Autodesk Fusion 360 part; units mm, degrees
(part 2 of 2)
  arc A365 (-6.1668, -296.7812) -> (-6.5328, -295.4151) centre (-7.0328, -296.2812) ccw
  arc A366 (-3.876, -300.2037) -> (-3.3, -299.7095) centre (-3.8, -299.7095) ccw
  line L347 (-6.6168, -297.5606) -> (-6.1668, -296.7812)
  arc A367 (-2.3, -290.7464) -> (-3.3, -291.7464) centre (-2.3, -291.7464) ccw
  line L348 (-3.6, -298.8464) -> (-4.55, -298.8464)
  arc A368 (-7.4653, -294.5303) -> (-7.3555, -294.9401) centre (-7.2055, -294.6803) ccw
  arc A369 (-5.55, -297.8464) -> (-4.55, -298.8464) centre (-4.55, -297.8464) ccw
  line L349 (-3.3, -291.7464) -> (-3.3, -295.7464)
  line L350 (-3.3, -299.1464) -> (-3.3, -299.7095)
  arc A370 (3.3, -291.7464) -> (2.3, -290.7464) centre (2.3, -291.7464) ccw
  line L351 (2.3, -290.7464) -> (-2.3, -290.7464)
  arc A371 (-3.6, -296.0464) -> (-3.3, -295.7464) centre (-3.6, -295.7464) ccw
  line L352 (-3.3, -299.1464) -> (-3.3, -295.7464)
  line L353 (3.3, -299.1464) -> (3.3, -299.7095)
  arc A372 (-5.5153, -291.1528) -> (-5.8814, -289.7868) centre (-6.3814, -290.6528) ccw
  arc A373 (-20.5017, -281.5828) -> (-21.8678, -281.2168) centre (-21.3678, -282.0828) ccw
  arc A374 (-23.8464, -279.55) -> (-22.8464, -280.55) centre (-22.8464, -279.55) ccw
  line L354 (-3.3, -254.3536) -> (-3.3, -258.2536)
  arc A375 (-3.3, -258.2536) -> (-2.3, -259.2536) centre (-2.3, -258.2536) ccw
  line L355 (-3.6, -251.1536) -> (-4.55, -251.1536)
  arc A376 (-23.765, -284.2451) -> (-23.0491, -284.4969) centre (-23.2991, -284.0639) ccw
  line L356 (3.3, -250.8536) -> (3.3, -250.2905)
  arc A377 (-5.8814, -260.2132) -> (-5.5153, -258.8472) centre (-6.3814, -259.3472) ccw
  line L357 (3.3, -258.2536) -> (3.3, -254.2536)
  arc A378 (-6.5828, -254.4983) -> (-6.2168, -253.1322) centre (-7.0828, -253.6322) ccw
  line L358 (-6.2168, -253.1322) -> (-6.6168, -252.4394)
  line L359 (-2.3, -259.2536) -> (2.3, -259.2536)
  arc A379 (3.3, -250.8536) -> (3.6, -251.1536) centre (3.6, -250.8536) ccw
  arc A380 (3.3, -299.7095) -> (3.876, -300.2037) centre (3.8, -299.7095) ccw
  line L360 (3.3, -250.8536) -> (3.3, -254.2536)
  line L361 (-7.4055, -254.9733) -> (-6.5828, -254.4983)
  arc A381 (-7.4055, -254.9733) -> (-7.5153, -255.3831) centre (-7.2555, -255.2331) ccw
  arc A382 (-3.6, -251.1536) -> (-3.3, -250.8536) centre (-3.6, -250.8536) ccw
  arc A383 (-4.55, -251.1536) -> (-5.55, -252.1536) centre (-4.55, -252.1536) ccw
  arc A384 (-3.3, -254.3536) -> (-3.6, -254.0536) centre (-3.6, -254.3536) ccw
  line L362 (-4.55, -254.0536) -> (-3.6, -254.0536)
  arc A385 (3.6, -253.9536) -> (3.3, -254.2536) centre (3.6, -254.2536) ccw
  line L363 (-3.3, -250.8536) -> (-3.3, -250.2905)
  line L364 (-17.0106, -291.2297) -> (-16.2312, -290.7797)
  arc A386 (-16.2297, -292.0106) -> (-15.8636, -293.3766) centre (-15.3636, -292.5106) ccw
  line L365 (-16.1528, -280.5153) -> (-19.6169, -282.5153)
  line L366 (-20.0267, -282.4055) -> (-20.5017, -281.5828)
  line L367 (-9.2153, -297.5614) -> (-9.4969, -298.0491)
  arc A387 (-19.889, -290.9586) -> (-15.9586, -294.889) centre (0, -275) ccw
  line L368 (-12.4868, -284.8651) -> (-14.7868, -280.8814)
  line L369 (-20.9464, -279.55) -> (-20.9464, -278.6)
  line L370 (-13.6409, -291.4268) -> (-14.4636, -290.9518)
  arc A388 (-22.5606, -281.6168) -> (-22.9266, -282.9828) centre (-22.0606, -282.4828) ccw
  arc A389 (-21.9464, -280.55) -> (-20.9464, -279.55) centre (-21.9464, -279.55) ccw
  line L371 (-24.1464, -278.3) -> (-20.6464, -278.3)
  arc A390 (-14.9311, -294.2614) -> (-15.0409, -293.8516) centre (-15.1909, -294.1114) ccw
  line L372 (-14.9311, -294.2614) -> (-13.2311, -291.3169)
  line L373 (-22.8464, -280.55) -> (-21.9464, -280.55)
  arc A391 (-19.7491, -290.2126) -> (-19.889, -290.9586) centre (-19.4991, -290.6457) ccw
  arc A392 (-13.6409, -291.4268) -> (-13.2311, -291.3169) centre (-13.4909, -291.1669) ccw
  arc A393 (-9.4969, -298.0491) -> (-9.2451, -298.765) centre (-9.0639, -298.2991) ccw
  arc A394 (-15.9586, -294.889) -> (-15.2126, -294.7491) centre (-15.6457, -294.4991) ccw
  line L374 (-16.2303, -288.1811) -> (-12.8528, -286.2311)
  arc A395 (-8.8055, -297.4516) -> (-9.2153, -297.5614) centre (-8.9555, -297.7114) ccw
  line L375 (-19.2614, -289.9311) -> (-19.7491, -290.2126)
  line L376 (-15.8297, -291.3178) -> (-16.2297, -292.0106)
  line L377 (-11.2311, -287.8528) -> (-13.2311, -291.3169)
  line L378 (-18.8516, -290.0409) -> (-18.3766, -290.8636)
  line L379 (-14.9311, -294.2614) -> (-15.2126, -294.7491)
  arc A396 (-18.3766, -290.8636) -> (-17.0106, -291.2297) centre (-17.5106, -290.3636) ccw
  arc A397 (-14.4636, -290.9518) -> (-15.8297, -291.3178) centre (-14.9636, -291.8178) ccw
  arc A398 (-16.2312, -290.7797) -> (-15.8651, -289.4136) centre (-16.7312, -289.9136) ccw
  arc A399 (-9.8651, -287.4868) -> (-11.2311, -287.8528) centre (-10.3651, -288.3528) ccw
  arc A400 (-16.2303, -288.1811) -> (-16.3401, -288.5909) centre (-16.0803, -288.4409) ccw
  line L380 (-15.0409, -293.8516) -> (-15.8636, -293.3766)
  line L381 (-15.8651, -289.4136) -> (-16.3401, -288.5909)
  arc A401 (-18.8516, -290.0409) -> (-19.2614, -289.9311) centre (-19.1114, -290.1909) ccw
  line L382 (-19.2614, -289.9311) -> (-16.2303, -288.1811)
  line L383 (-20.4151, -268.4672) -> (-19.9401, -267.6445)
  line L384 (-23.8464, -271.4) -> (-23.8464, -270.45)
  line L385 (-22.0464, -269.45) -> (-22.8464, -269.45)
  arc A402 (-22.9266, -267.0172) -> (-22.5606, -268.3832) centre (-22.0606, -267.5172) ccw
  arc A403 (-21.7812, -268.8332) -> (-20.4151, -268.4672) centre (-21.2812, -267.9672) ccw
  line L386 (-14.7868, -269.1186) -> (-12.4868, -265.1349)
  arc A404 (-19.5303, -267.5347) -> (-19.9401, -267.6445) centre (-19.6803, -267.7945) ccw
  arc A405 (-22.4516, -266.1945) -> (-22.5614, -265.7847) centre (-22.7114, -266.0445) ccw
  arc A406 (-12.4868, -265.1349) -> (-12.8528, -263.7689) centre (-13.3528, -264.6349) ccw
  line L387 (-19.5303, -267.5347) -> (-16.1528, -269.4847)
  arc A407 (-21.0464, -270.45) -> (-22.0464, -269.45) centre (-22.0464, -270.45) ccw
  line L388 (-24.1464, -271.7) -> (-24.7095, -271.7)
  line L389 (-22.5606, -268.3832) -> (-21.7812, -268.8332)
  line L390 (-22.4516, -266.1945) -> (-22.9266, -267.0172)
  line L391 (-24.1464, -271.7) -> (-20.7464, -271.7)
  arc A408 (-23.765, -265.7549) -> (-25.2037, -271.124) centre (0, -275) ccw
  arc A409 (-16.1528, -269.4847) -> (-14.7868, -269.1186) centre (-15.6528, -268.6186) ccw
  line L392 (-16.7464, -271.7) -> (-20.7464, -271.7)
  arc A410 (-22.8464, -269.45) -> (-23.8464, -270.45) centre (-22.8464, -270.45) ccw
  arc A411 (-21.0464, -271.4) -> (-20.7464, -271.7) centre (-20.7464, -271.4) ccw
  line L393 (-21.0464, -271.4) -> (-21.0464, -270.45)
  arc A412 (-25.2037, -271.124) -> (-24.7095, -271.7) centre (-24.7095, -271.2) ccw
  arc A413 (-15.7464, -272.7) -> (-16.7464, -271.7) centre (-16.7464, -272.7) ccw
  arc A414 (-24.1464, -271.7) -> (-23.8464, -271.4) centre (-24.1464, -271.4) ccw
  arc A415 (-23.0491, -265.5031) -> (-23.765, -265.7549) centre (-23.2991, -265.9361) ccw
  line L394 (-22.5614, -265.7847) -> (-23.0491, -265.5031)
  line L395 (-22.5614, -265.7847) -> (-19.5303, -267.5347)
  line L396 (16.7464, -278.3) -> (20.7464, -278.3)
  line L397 (21.0464, -278.6) -> (21.0464, -279.55)
  line L398 (22.5614, -284.2153) -> (19.5303, -282.4653)
  arc A416 (23.0491, -284.4969) -> (23.765, -284.2451) centre (23.2991, -284.0639) ccw
  line L399 (23.8464, -278.6) -> (23.8464, -279.55)
  line L400 (14.7868, -280.8814) -> (12.4868, -284.8651)
  arc A417 (21.7812, -281.1668) -> (20.4151, -281.5328) centre (21.2812, -282.0328) ccw
  arc A418 (12.4868, -284.8651) -> (12.8528, -286.2311) centre (13.3528, -285.3651) ccw
  arc A419 (22.9266, -282.9828) -> (22.5606, -281.6168) centre (22.0606, -282.4828) ccw
  arc A420 (19.5303, -282.4653) -> (19.9401, -282.3555) centre (19.6803, -282.2055) ccw
  arc A421 (24.1464, -278.3) -> (23.8464, -278.6) centre (24.1464, -278.6) ccw
  arc A422 (23.765, -284.2451) -> (25.2037, -278.876) centre (0, -275) ccw
  arc A423 (16.1528, -280.5153) -> (14.7868, -280.8814) centre (15.6528, -281.3814) ccw
  arc A424 (5.55, -252.1536) -> (4.55, -251.1536) centre (4.55, -252.1536) ccw
  arc A425 (-16.4267, -261.3591) -> (-16.3169, -261.7689) centre (-16.1669, -261.5091) ccw
  line L401 (-16.4267, -261.3591) -> (-15.9517, -260.5364)
  line L402 (8.8055, -252.5484) -> (7.9828, -252.0734)
  line L403 (-9.2153, -252.4386) -> (-9.4969, -251.9509)
  arc A426 (-11.2311, -262.1472) -> (-9.8651, -262.5132) centre (-10.3651, -261.6472) ccw
  line L404 (5.5153, -291.1528) -> (7.5153, -294.6169)
  arc A427 (-15.9586, -255.111) -> (-19.889, -259.0414) centre (0, -275) ccw
  line L405 (7.4055, -295.0268) -> (6.5828, -295.5018)
  arc A428 (-17.0106, -258.7703) -> (-18.3766, -259.1364) centre (-17.5106, -259.6364) ccw
  arc A429 (6.6168, -297.5606) -> (7.9828, -297.9266) centre (7.4828, -297.0606) ccw
  arc A430 (-15.8636, -256.6234) -> (-16.2297, -257.9894) centre (-15.3636, -257.4894) ccw
  line L406 (-14.9311, -255.7386) -> (-13.1811, -258.7697)
  line L407 (9.2153, -297.5614) -> (7.5153, -294.6169)
  line L408 (-15.0409, -256.1484) -> (-15.8636, -256.6234)
  arc A431 (9.4969, -251.9509) -> (9.2451, -251.235) centre (9.0639, -251.7009) ccw
  line L409 (-18.8516, -259.9591) -> (-18.3766, -259.1364)
  arc A432 (-15.7797, -258.7688) -> (-14.4136, -259.1349) centre (-14.9136, -258.2688) ccw
  arc A433 (-15.2126, -255.2509) -> (-15.9586, -255.111) centre (-15.6457, -255.5009) ccw
  line L410 (-16.3178, -259.1703) -> (-17.0106, -258.7703)
  arc A434 (7.4055, -295.0268) -> (7.5153, -294.6169) centre (7.2555, -294.7669) ccw
  arc A435 (-9.2153, -252.4386) -> (-8.8055, -252.5484) centre (-8.9555, -252.2886) ccw
  line L411 (5.55, -252.9536) -> (5.55, -252.1536)
  line L412 (-14.9311, -255.7386) -> (-15.2126, -255.2509)
  arc A436 (-13.1811, -258.7697) -> (-13.5909, -258.6599) centre (-13.4409, -258.9197) ccw
  arc A437 (-19.2614, -260.0689) -> (-18.8516, -259.9591) centre (-19.1114, -259.8091) ccw
  line L413 (9.2153, -252.4386) -> (7.4653, -255.4697)
  line L414 (5.8814, -260.2132) -> (9.8651, -262.5132)
  line L415 (-19.2614, -260.0689) -> (-16.3169, -261.7689)
  arc A438 (5.8814, -289.7868) -> (5.5153, -291.1528) centre (6.3814, -290.6528) ccw
  line L416 (-9.8651, -262.5132) -> (-5.8814, -260.2132)
  line L417 (-8.8055, -252.5484) -> (-7.9828, -252.0734)
  arc A439 (6.1668, -253.2188) -> (6.5328, -254.5849) centre (7.0328, -253.7188) ccw
  line L418 (-5.8814, -289.7868) -> (-9.8651, -287.4868)
  arc A440 (11.2311, -287.8528) -> (9.8651, -287.4868) centre (10.3651, -288.3528) ccw
  line L419 (9.2153, -252.4386) -> (9.4969, -251.9509)
  line L420 (-16.2297, -257.9894) -> (-15.7797, -258.7688)
  line L421 (9.8651, -287.4868) -> (5.8814, -289.7868)
  arc A441 (9.2153, -297.5614) -> (8.8055, -297.4516) centre (8.9555, -297.7114) ccw
  arc A442 (5.55, -296.9464) -> (4.55, -295.9464) centre (4.55, -296.9464) ccw
  line L422 (-12.8528, -263.7689) -> (-16.3169, -261.7689)
  line L423 (6.2168, -296.8678) -> (6.6168, -297.5606)
  line L424 (-14.4136, -259.1349) -> (-13.5909, -258.6599)
  arc A443 (-15.0409, -256.1484) -> (-14.9311, -255.7386) centre (-15.1909, -255.8886) ccw
  arc A444 (-19.889, -259.0414) -> (-19.7491, -259.7874) centre (-19.4991, -259.3544) ccw
  line L425 (7.4653, -255.4697) -> (5.5153, -258.8472)
  arc A445 (-15.9517, -260.5364) -> (-16.3178, -259.1703) centre (-16.8178, -260.0364) ccw
  arc A446 (7.4653, -255.4697) -> (7.3555, -255.0599) centre (7.2055, -255.3197) ccw
  line L426 (4.55, -295.9464) -> (3.6, -295.9464)
  line L427 (-9.2153, -252.4386) -> (-7.5153, -255.3831)
  line L428 (-8.8055, -297.4516) -> (-7.9828, -297.9266)
  line L429 (-15.7464, -277.3) -> (-15.7464, -272.7)
  arc A447 (9.2451, -298.765) -> (9.4969, -298.0491) centre (9.0639, -298.2991) ccw
  arc A448 (-9.2451, -251.235) -> (-9.4969, -251.9509) centre (-9.0639, -251.7009) ccw
  arc A449 (3.876, -300.2037) -> (9.2451, -298.765) centre (0, -275) ccw
  arc A450 (-9.2451, -298.765) -> (-3.876, -300.2037) centre (0, -275) ccw
  arc A451 (7.9828, -252.0734) -> (6.6168, -252.4394) centre (7.4828, -252.9394) ccw
  arc A452 (8.8055, -252.5484) -> (9.2153, -252.4386) centre (8.9555, -252.2886) ccw
  arc A453 (-3.876, -249.7963) -> (-9.2451, -251.235) centre (0, -275) ccw
  line L430 (-9.2153, -297.5614) -> (-7.4653, -294.5303)
  line L431 (-13.1811, -258.7697) -> (-11.2311, -262.1472)
  line L432 (-19.2614, -260.0689) -> (-19.7491, -259.7874)
  arc A454 (5.5153, -258.8472) -> (5.8814, -260.2132) centre (6.3814, -259.3472) ccw
  line L433 (6.5328, -254.5849) -> (7.3555, -255.0599)
  line L434 (6.6168, -252.4394) -> (6.1668, -253.2188)
  arc A455 (9.8651, -262.5132) -> (11.2311, -262.1472) centre (10.3651, -261.6472) ccw
  arc A456 (4.55, -298.8464) -> (5.55, -297.8464) centre (4.55, -297.8464) ccw
  line L435 (3.6, -298.8464) -> (4.55, -298.8464)
  arc A457 (4.55, -253.9536) -> (5.55, -252.9536) centre (4.55, -252.9536) ccw
  line L436 (3.6, -251.1536) -> (4.55, -251.1536)
  arc A458 (6.5828, -295.5018) -> (6.2168, -296.8678) centre (7.0828, -296.3678) ccw
  line L437 (8.8055, -297.4516) -> (7.9828, -297.9266)
  line L438 (9.2153, -297.5614) -> (9.4969, -298.0491)
  line L439 (5.55, -297.8464) -> (5.55, -296.9464)
  arc A459 (9.2451, -251.235) -> (3.876, -249.7963) centre (0, -275) ccw
  line L440 (3.6, -253.9536) -> (4.55, -253.9536)
  arc A460 (25.2037, -278.876) -> (24.7095, -278.3) centre (24.7095, -278.8) ccw
  line L441 (22.0464, -280.55) -> (22.8464, -280.55)
  line L442 (19.5303, -282.4653) -> (16.1528, -280.5153)
  line L443 (24.1464, -278.3) -> (24.7095, -278.3)
  arc A461 (22.8464, -280.55) -> (23.8464, -279.55) centre (22.8464, -279.55) ccw
  line L444 (24.1464, -278.3) -> (20.7464, -278.3)
  line L445 (22.5614, -284.2153) -> (23.0491, -284.4969)
  line L446 (20.4151, -281.5328) -> (19.9401, -282.3555)
  arc A462 (21.0464, -278.6) -> (20.7464, -278.3) centre (20.7464, -278.6) ccw
  arc A463 (22.4516, -283.8055) -> (22.5614, -284.2153) centre (22.7114, -283.9555) ccw
  arc A464 (21.0464, -279.55) -> (22.0464, -280.55) centre (22.0464, -279.55) ccw
  line L447 (22.5606, -281.6168) -> (21.7812, -281.1668)
  arc A465 (15.7464, -277.3) -> (16.7464, -278.3) centre (16.7464, -277.3) ccw
  line L448 (22.4516, -283.8055) -> (22.9266, -282.9828)
  arc A466 (17.0106, -291.2297) -> (18.3766, -290.8636) centre (17.5106, -290.3636) ccw
  line L449 (18.8516, -259.9591) -> (18.3766, -259.1364)
  line L450 (15.0409, -293.8516) -> (15.8636, -293.3766)
  arc A467 (15.8636, -293.3766) -> (16.2297, -292.0106) centre (15.3636, -292.5106) ccw
  line L451 (23.8464, -271.4) -> (23.8464, -270.45)
  line L452 (15.0409, -256.1484) -> (15.8636, -256.6234)
  arc A468 (15.2126, -294.7491) -> (15.9586, -294.889) centre (15.6457, -294.4991) ccw
  arc A469 (22.5614, -265.7847) -> (22.4516, -266.1945) centre (22.7114, -266.0445) ccw
  arc A470 (19.889, -290.9586) -> (19.7491, -290.2126) centre (19.4991, -290.6457) ccw
  line L453 (19.2614, -289.9311) -> (16.3169, -288.2311)
  arc A471 (20.6464, -271.7) -> (20.9464, -271.4) centre (20.6464, -271.4) ccw
  arc A472 (16.4267, -288.6409) -> (16.3169, -288.2311) centre (16.1669, -288.4909) ccw
  arc A473 (15.7797, -291.2312) -> (14.4136, -290.8651) centre (14.9136, -291.7312) ccw
  arc A474 (15.9586, -255.111) -> (15.2126, -255.2509) centre (15.6457, -255.5009) ccw
  line L454 (14.4136, -290.8651) -> (13.5909, -291.3401)
  arc A475 (13.1811, -291.2303) -> (13.5909, -291.3401) centre (13.4409, -291.0803) ccw
  arc A476 (19.2614, -289.9311) -> (18.8516, -290.0409) centre (19.1114, -290.1909) ccw
  line L455 (13.1811, -291.2303) -> (11.2311, -287.8528)
  line L456 (12.8528, -286.2311) -> (16.3169, -288.2311)
  line L457 (16.3178, -290.8297) -> (17.0106, -291.2297)
  line L458 (16.2303, -261.8189) -> (12.8528, -263.7689)
  arc A477 (25.2037, -271.124) -> (23.765, -265.7549) centre (0, -275) ccw
  line L459 (14.9311, -294.2614) -> (15.2126, -294.7491)
  arc A478 (20.5017, -268.4172) -> (21.8678, -268.7832) centre (21.3678, -267.9172) ccw
  line L460 (19.2614, -289.9311) -> (19.7491, -290.2126)
  line L461 (14.9311, -294.2614) -> (13.1811, -291.2303)
  line L462 (15.7464, -272.7) -> (15.7464, -277.3)
  line L463 (16.4267, -288.6409) -> (15.9517, -289.4636)
  line L464 (18.8516, -290.0409) -> (18.3766, -290.8636)
  line L465 (21.8678, -268.7832) -> (22.5606, -268.3832)
  line L466 (16.2297, -292.0106) -> (15.7797, -291.2312)
  line L467 (20.0267, -267.5945) -> (20.5017, -268.4172)
  arc A479 (23.8464, -270.45) -> (22.8464, -269.45) centre (22.8464, -270.45) ccw
  arc A480 (15.9586, -294.889) -> (19.889, -290.9586) centre (0, -275) ccw
  arc A481 (14.7868, -269.1186) -> (16.1528, -269.4847) centre (15.6528, -268.6186) ccw
  arc A482 (18.8516, -259.9591) -> (19.2614, -260.0689) centre (19.1114, -259.8091) ccw
  arc A483 (23.8464, -271.4) -> (24.1464, -271.7) centre (24.1464, -271.4) ccw
  arc A484 (15.9517, -289.4636) -> (16.3178, -290.8297) centre (16.8178, -289.9636) ccw
  line L468 (17.0106, -258.7703) -> (16.2312, -259.2203)
  arc A485 (22.5606, -268.3832) -> (22.9266, -267.0172) centre (22.0606, -267.5172) ccw
  line L469 (15.8651, -260.5864) -> (16.3401, -261.4091)
  arc A486 (12.8528, -263.7689) -> (12.4868, -265.1349) centre (13.3528, -264.6349) ccw
  line L470 (11.2311, -262.1472) -> (13.2311, -258.6831)
  line L471 (20.6464, -271.7) -> (16.7464, -271.7)
  line L472 (24.1464, -271.7) -> (20.6464, -271.7)
  line L473 (20.9464, -270.45) -> (20.9464, -271.4)
  line L474 (22.5614, -265.7847) -> (23.0491, -265.5031)
  line L475 (14.9311, -255.7386) -> (15.2126, -255.2509)
  line L476 (22.5614, -265.7847) -> (19.6169, -267.4847)
  arc A487 (16.2303, -261.8189) -> (16.3401, -261.4091) centre (16.0803, -261.5591) ccw
  line L477 (16.1528, -269.4847) -> (19.6169, -267.4847)
  arc A488 (19.889, -259.0414) -> (15.9586, -255.111) centre (0, -275) ccw
  arc A489 (21.9464, -269.45) -> (20.9464, -270.45) centre (21.9464, -270.45) ccw
  arc A490 (15.0409, -293.8516) -> (14.9311, -294.2614) centre (15.1909, -294.1114) ccw
  line L478 (13.6409, -258.5733) -> (14.4636, -259.0483)
  line L479 (12.4868, -265.1349) -> (14.7868, -269.1186)
  line L480 (22.8464, -269.45) -> (21.9464, -269.45)
  arc A491 (18.3766, -259.1364) -> (17.0106, -258.7703) centre (17.5106, -259.6364) ccw
  arc A492 (16.2297, -257.9894) -> (15.8636, -256.6234) centre (15.3636, -257.4894) ccw
  line L481 (19.2614, -260.0689) -> (19.7491, -259.7874)
  arc A493 (14.9311, -255.7386) -> (15.0409, -256.1484) centre (15.1909, -255.8886) ccw
  arc A494 (13.6409, -258.5733) -> (13.2311, -258.6831) centre (13.4909, -258.8331) ccw
  line L482 (22.4516, -266.1945) -> (22.9266, -267.0172)
  arc A495 (14.4636, -259.0483) -> (15.8297, -258.6822) centre (14.9636, -258.1822) ccw
  arc A496 (20.0267, -267.5945) -> (19.6169, -267.4847) centre (19.7669, -267.7445) ccw
  line L483 (24.1464, -271.7) -> (24.7095, -271.7)
  arc A497 (16.2312, -259.2203) -> (15.8651, -260.5864) centre (16.7312, -260.0864) ccw
  line L484 (14.9311, -255.7386) -> (13.2311, -258.6831)
  arc A498 (23.765, -265.7549) -> (23.0491, -265.5031) centre (23.2991, -265.9361) ccw
  line L485 (19.2614, -260.0689) -> (16.2303, -261.8189)
  line L486 (15.8297, -258.6822) -> (16.2297, -257.9894)
  arc A499 (19.7491, -259.7874) -> (19.889, -259.0414) centre (19.4991, -259.3544) ccw
  arc A500 (16.7464, -271.7) -> (15.7464, -272.7) centre (16.7464, -272.7) ccw
  arc A501 (24.7095, -271.7) -> (25.2037, -271.124) centre (24.7095, -271.2) ccw
  circle A502 centre (0, -210) radius 10.7464
  circle A503 centre (0, -223.2464) radius 1.5
  circle A504 centre (11.4718, -216.6232) radius 1.5
  circle A505 centre (11.4718, -203.3768) radius 1.5
  circle A506 centre (0, -196.7536) radius 1.5
  circle A507 centre (-11.4718, -203.3768) radius 1.5
  circle A508 centre (-11.4718, -216.6232) radius 1.5
  circle A509 centre (0, -275) radius 10.7464
  circle A510 centre (0, -288.2464) radius 1.5
  circle A511 centre (11.4718, -281.6232) radius 1.5
  circle A512 centre (11.4718, -268.3768) radius 1.5
  circle A513 centre (0, -261.7536) radius 1.5
  circle A514 centre (-11.4718, -268.3768) radius 1.5
  circle A515 centre (-11.4718, -281.6232) radius 1.5
  dimension "d2" = 1
  dimension "d3" = 1
  dimension "d4" = 1
  dimension "d5" = 1
  dimension "d6" = 1
  dimension "d7" = 1
  dimension "d8" = 0.3
  dimension "d9" = 0.3
  dimension "d10" = 0.3
  dimension "d11" = 0.3
  dimension "d12" = 0.5
  dimension "d13" = 0.5
  dimension "d15" = 360
  dimension "d17" = 360
  dimension "d23" = 360
  dimension "d25" = 360
  dimension "d26" = 1
  dimension "d27" = 1
  dimension "d28" = 1
  dimension "d29" = 1
  dimension "d30" = 1
  dimension "d31" = 1
  dimension "d32" = 0.3
  dimension "d33" = 0.3
  dimension "d34" = 0.3
  dimension "d35" = 0.3
  dimension "d36" = 0.5
  dimension "d37" = 0.5
  dimension "d41" = 3
  dimension "d43" = 360
  dimension "d45" = 3
  dimension "d47" = 360
  constraint perpendicular L43 L152
  constraint coincident L44.end A61.start
  constraint parallel L44 L153
  constraint coincident A50.end L34.start
  constraint parallel L34 L154
  constraint parallel L44 L155
  constraint coincident L43.end A60.start
  constraint tangent A60 L156
  constraint tangent A60 L157
  constraint coincident L42.end A59.end
  constraint tangent A59 L158
  constraint tangent A59 L159
  constraint coincident L41.end A58.end
  constraint tangent A58 L160
  constraint tangent A58 L161
  constraint coincident L40.end A57.start
  constraint tangent A57 L162
  constraint tangent A57 L163
  constraint coincident L39.end A56.end
  constraint tangent A56 L164
  constraint tangent A56 L165
  constraint coincident L38.end A55.end
  constraint tangent A55 L166
  constraint tangent A55 L167
  constraint midpoint L37 L168.start
  constraint perpendicular L167 L168
  constraint parallel L37 L169
  constraint coincident L36.end A53.end
  constraint tangent A53 L170
  constraint tangent A53 L171
  constraint coincident L35.end A52.end
  constraint tangent A52 L172
  constraint tangent A52 L173
  constraint perpendicular L173 L174
  constraint perpendicular L184 L185
  constraint perpendicular L180 L184
  constraint perpendicular L177 L178
  constraint perpendicular L177 L179
  constraint perpendicular L175 L176
  constraint tangent L176 A190
  constraint tangent L175 A190
  constraint tangent L175 A191
  constraint tangent L183 A191
  constraint tangent L177 A192
  constraint tangent L178 A192
  constraint tangent L182 A193
  constraint tangent L178 A193
  constraint tangent L185 A194
  constraint tangent L184 A194
  constraint tangent L184 A195
  constraint tangent L180 A195
  constraint tangent L183 A196
  constraint tangent L185 A196
  constraint tangent L176 A197
  constraint tangent L181 A197
  constraint tangent L179 A198
  constraint tangent L177 A198
  constraint tangent L182 A199
  constraint tangent L180 A199
  constraint tangent A200 A334
  constraint tangent L181 A200
  constraint tangent L179 A201
  constraint tangent A201 A334
  constraint concentric A334 A335
  constraint concentric A335 A336
  constraint concentric A336 A337
  constraint concentric A337 A338
  constraint concentric A338 A339
  constraint concentric A339 A340
  constraint concentric A340 A341
  constraint concentric A341 A342
  constraint concentric A342 A343
  constraint concentric A343 A344
  constraint concentric A344 A345
  constraint tangent A196 L307
  constraint tangent A199 L308
  constraint perpendicular L345 L351
  constraint perpendicular L349 L351
  constraint perpendicular L339 L348
  constraint perpendicular L348 L350
  constraint perpendicular L435 L439
  constraint tangent A456 L435
  constraint tangent A456 L439
  constraint tangent A442 L439
  constraint tangent A442 L426
  constraint tangent L348 A369
  constraint tangent L339 A369
  constraint tangent A355 L344
  constraint tangent A355 L339
  constraint tangent L345 A370
  constraint tangent A370 L351
  constraint tangent A367 L351
  constraint tangent A367 L349
  constraint tangent A362 L426
  constraint tangent A362 L345
  constraint tangent A359 L435
  constraint tangent A359 L353
  constraint tangent A363 L350
  constraint tangent A363 L348
  constraint tangent L344 A371
  constraint tangent L349 A371
  constraint tangent A380 A449
  constraint tangent L353 A380
  constraint tangent A366 L350
  constraint tangent A366 A449
  constraint concentric A449 A480
  constraint concentric A422 A480
  constraint concentric A422 A477
  constraint concentric A477 A488
  constraint concentric A459 A488
  constraint concentric A453 A459
  constraint concentric A427 A453
  constraint concentric A408 A427
  constraint concentric A350 A408
  constraint concentric A350 A387
  constraint concentric A387 A450
  constraint tangent A362 L346
  constraint tangent A371 L352
  measures "d2" radius of A190
  measures "d3" radius of A191
  measures "d4" radius of A192
  measures "d5" radius of A193
  measures "d6" radius of A194
  measures "d7" radius of A195
  measures "d8" radius of A196
  measures "d9" radius of A197
  measures "d10" radius of A198
  measures "d11" radius of A199
  measures "d12" radius of A200
  measures "d13" radius of A201
  measures "d26" radius of A456
  measures "d27" radius of A442
  measures "d28" radius of A369
  measures "d29" radius of A355
  measures "d30" radius of A370
  measures "d31" radius of A367
  measures "d32" radius of A362
  measures "d33" radius of A359
  measures "d34" radius of A363
  measures "d35" radius of A371
  measures "d36" radius of A380
  measures "d37" radius of A366
  measures "d41" diameter of A503
  measures "d45" diameter of A510
sketch "スケッチ2" plane through (0, 3, 0) normal (0, 1, 0) x (-1, 0, 0)
  circle A0 centre (-11.4718, 6.6232) radius 1.5
  circle A1 centre (0, 0) radius 10.7464
  circle A2 centre (-11.4718, -6.6232) radius 1.5
  circle A3 centre (11.4718, -6.6232) radius 1.5
  circle A4 centre (0, 13.2464) radius 1.5
  circle A5 centre (11.4718, 6.6232) radius 1.5
  circle A6 centre (0, -13.2464) radius 1.5
  line L0 (9.4969, -23.0491) -> (5.5153, -16.1528)
  arc A7 (5.8814, -14.7868) -> (5.5153, -16.1528) centre (6.3814, -15.6528) ccw
  line L1 (5.8814, -14.7868) -> (9.8651, -12.4868)
  arc A8 (11.2311, -12.8528) -> (9.8651, -12.4868) centre (10.3651, -13.3528) ccw
  line L2 (11.2311, -12.8528) -> (15.2126, -19.7491)
  arc A9 (15.2126, -19.7491) -> (15.9586, -19.889) centre (15.6457, -19.4991) ccw
  arc A10 (15.9586, -19.889) -> (19.889, -15.9586) centre (0, 0) ccw
  arc A11 (19.889, -15.9586) -> (19.7491, -15.2126) centre (19.4991, -15.6457) ccw
  line L3 (19.7491, -15.2126) -> (12.8528, -11.2311)
  arc A12 (12.4868, -9.8651) -> (12.8528, -11.2311) centre (13.3528, -10.3651) ccw
  line L4 (12.4868, -9.8651) -> (14.7868, -5.8814)
  arc A13 (16.1528, -5.5153) -> (14.7868, -5.8814) centre (15.6528, -6.3814) ccw
  line L5 (16.1528, -5.5153) -> (23.0491, -9.4969)
  arc A14 (23.0491, -9.4969) -> (23.765, -9.2451) centre (23.2991, -9.0639) ccw
  arc A15 (23.765, -9.2451) -> (25.2037, -3.876) centre (0, 0) ccw
  arc A16 (25.2037, -3.876) -> (24.7095, -3.3) centre (24.7095, -3.8) ccw
  line L6 (24.7095, -3.3) -> (16.7464, -3.3)
  arc A17 (15.7464, -2.3) -> (16.7464, -3.3) centre (16.7464, -2.3) ccw
  line L7 (15.7464, -2.3) -> (15.7464, 2.3)
  arc A18 (16.7464, 3.3) -> (15.7464, 2.3) centre (16.7464, 2.3) ccw
  line L8 (16.7464, 3.3) -> (24.7095, 3.3)
  arc A19 (24.7095, 3.3) -> (25.2037, 3.876) centre (24.7095, 3.8) ccw
  arc A20 (25.2037, 3.876) -> (23.765, 9.2451) centre (0, 0) ccw
  arc A21 (23.765, 9.2451) -> (23.0491, 9.4969) centre (23.2991, 9.0639) ccw
  line L9 (23.0491, 9.4969) -> (16.1528, 5.5153)
  arc A22 (14.7868, 5.8814) -> (16.1528, 5.5153) centre (15.6528, 6.3814) ccw
  line L10 (14.7868, 5.8814) -> (12.4868, 9.8651)
  arc A23 (12.8528, 11.2311) -> (12.4868, 9.8651) centre (13.3528, 10.3651) ccw
  line L11 (12.8528, 11.2311) -> (19.7491, 15.2126)
  arc A24 (19.7491, 15.2126) -> (19.889, 15.9586) centre (19.4991, 15.6457) ccw
  arc A25 (19.889, 15.9586) -> (15.9586, 19.889) centre (0, 0) ccw
  arc A26 (15.9586, 19.889) -> (15.2126, 19.7491) centre (15.6457, 19.4991) ccw
  line L12 (15.2126, 19.7491) -> (11.2311, 12.8528)
  arc A27 (9.8651, 12.4868) -> (11.2311, 12.8528) centre (10.3651, 13.3528) ccw
  line L13 (9.8651, 12.4868) -> (5.8814, 14.7868)
  arc A28 (5.5153, 16.1528) -> (5.8814, 14.7868) centre (6.3814, 15.6528) ccw
  line L14 (5.5153, 16.1528) -> (9.4969, 23.0491)
  arc A29 (9.4969, 23.0491) -> (9.2451, 23.765) centre (9.0639, 23.2991) ccw
  arc A30 (9.2451, 23.765) -> (3.876, 25.2037) centre (0, 0) ccw
  arc A31 (3.876, 25.2037) -> (3.3, 24.7095) centre (3.8, 24.7095) ccw
  line L15 (3.3, 24.7095) -> (3.3, 16.7464)
  arc A32 (2.3, 15.7464) -> (3.3, 16.7464) centre (2.3, 16.7464) ccw
  line L16 (2.3, 15.7464) -> (-2.3, 15.7464)
  arc A33 (-3.3, 16.7464) -> (-2.3, 15.7464) centre (-2.3, 16.7464) ccw
  line L17 (-3.3, 16.7464) -> (-3.3, 24.7095)
  arc A34 (-3.3, 24.7095) -> (-3.876, 25.2037) centre (-3.8, 24.7095) ccw
  arc A35 (-3.876, 25.2037) -> (-9.2451, 23.765) centre (0, 0) ccw
  arc A36 (-9.2451, 23.765) -> (-9.4969, 23.0491) centre (-9.0639, 23.2991) ccw
  line L18 (-9.4969, 23.0491) -> (-5.5153, 16.1528)
  arc A37 (-5.8814, 14.7868) -> (-5.5153, 16.1528) centre (-6.3814, 15.6528) ccw
  line L19 (-5.8814, 14.7868) -> (-9.8651, 12.4868)
  arc A38 (-11.2311, 12.8528) -> (-9.8651, 12.4868) centre (-10.3651, 13.3528) ccw
  line L20 (-11.2311, 12.8528) -> (-15.2126, 19.7491)
  arc A39 (-15.2126, 19.7491) -> (-15.9586, 19.889) centre (-15.6457, 19.4991) ccw
  arc A40 (-15.9586, 19.889) -> (-19.889, 15.9586) centre (0, 0) ccw
  arc A41 (-19.889, 15.9586) -> (-19.7491, 15.2126) centre (-19.4991, 15.6457) ccw
  line L21 (-19.7491, 15.2126) -> (-12.8528, 11.2311)
  arc A42 (-12.4868, 9.8651) -> (-12.8528, 11.2311) centre (-13.3528, 10.3651) ccw
  line L22 (-12.4868, 9.8651) -> (-14.7868, 5.8814)
  arc A43 (-16.1528, 5.5153) -> (-14.7868, 5.8814) centre (-15.6528, 6.3814) ccw
  line L23 (-16.1528, 5.5153) -> (-23.0491, 9.4969)
  arc A44 (-23.0491, 9.4969) -> (-23.765, 9.2451) centre (-23.2991, 9.0639) ccw
  arc A45 (-23.765, 9.2451) -> (-25.2037, 3.876) centre (0, 0) ccw
  arc A46 (-25.2037, 3.876) -> (-24.7095, 3.3) centre (-24.7095, 3.8) ccw
  line L24 (-24.7095, 3.3) -> (-16.7464, 3.3)
  arc A47 (-15.7464, 2.3) -> (-16.7464, 3.3) centre (-16.7464, 2.3) ccw
  line L25 (-15.7464, 2.3) -> (-15.7464, -2.3)
  arc A48 (-16.7464, -3.3) -> (-15.7464, -2.3) centre (-16.7464, -2.3) ccw
  line L26 (-16.7464, -3.3) -> (-24.7095, -3.3)
  arc A49 (-24.7095, -3.3) -> (-25.2037, -3.876) centre (-24.7095, -3.8) ccw
  arc A50 (-25.2037, -3.876) -> (-23.765, -9.2451) centre (0, 0) ccw
  arc A51 (-23.765, -9.2451) -> (-23.0491, -9.4969) centre (-23.2991, -9.0639) ccw
  line L27 (-23.0491, -9.4969) -> (-16.1528, -5.5153)
  arc A52 (-14.7868, -5.8814) -> (-16.1528, -5.5153) centre (-15.6528, -6.3814) ccw
  line L28 (-14.7868, -5.8814) -> (-12.4868, -9.8651)
  arc A53 (-12.8528, -11.2311) -> (-12.4868, -9.8651) centre (-13.3528, -10.3651) ccw
  line L29 (-12.8528, -11.2311) -> (-19.7491, -15.2126)
  arc A54 (-19.7491, -15.2126) -> (-19.889, -15.9586) centre (-19.4991, -15.6457) ccw
  arc A55 (-19.889, -15.9586) -> (-15.9586, -19.889) centre (0, 0) ccw
  arc A56 (-15.9586, -19.889) -> (-15.2126, -19.7491) centre (-15.6457, -19.4991) ccw
  line L30 (-15.2126, -19.7491) -> (-11.2311, -12.8528)
  arc A57 (-9.8651, -12.4868) -> (-11.2311, -12.8528) centre (-10.3651, -13.3528) ccw
  line L31 (-9.8651, -12.4868) -> (-5.8814, -14.7868)
  arc A58 (-5.5153, -16.1528) -> (-5.8814, -14.7868) centre (-6.3814, -15.6528) ccw
  line L32 (-5.5153, -16.1528) -> (-9.4969, -23.0491)
  arc A59 (-9.4969, -23.0491) -> (-9.2451, -23.765) centre (-9.0639, -23.2991) ccw
  arc A60 (-9.2451, -23.765) -> (-3.876, -25.2037) centre (0, 0) ccw
  arc A61 (-3.876, -25.2037) -> (-3.3, -24.7095) centre (-3.8, -24.7095) ccw
  line L33 (-3.3, -24.7095) -> (-3.3, -16.7464)
  arc A62 (-2.3, -15.7464) -> (-3.3, -16.7464) centre (-2.3, -16.7464) ccw
  line L34 (-2.3, -15.7464) -> (2.3, -15.7464)
  arc A63 (3.3, -16.7464) -> (2.3, -15.7464) centre (2.3, -16.7464) ccw
  line L35 (3.3, -16.7464) -> (3.3, -24.7095)
  arc A64 (3.3, -24.7095) -> (3.876, -25.2037) centre (3.8, -24.7095) ccw
  arc A65 (3.876, -25.2037) -> (9.2451, -23.765) centre (0, 0) ccw
  arc A66 (9.2451, -23.765) -> (9.4969, -23.0491) centre (9.0639, -23.2991) ccw
  line L36 (-6.0822, -22.6993) -> (-5.6959, -22.8028)
  line L37 (-6.0822, -22.6993) -> (-6.4686, -22.5957)
  line L38 (-5.6959, -22.8028) -> (-2.9767, -12.6546)
  line L39 (-6.4686, -22.5957) -> (-3.7494, -12.4476)
  line L40 (-2.9767, -12.6546) -> (-3.7494, -12.4476)
  dimension "d63" = 0.4
  dimension "d64" = 0.4
  constraint perpendicular L39 L40
  measures "d63" distance of L36.start L36.end
  measures "d64" distance of L36.start L37.end
sketch "スケッチ3" plane through (0.3864, 0, 0.1035) normal (0.965926, 0, 0.258819) x (0.258819, 0, -0.965926)
  line L0 (23.5, 3) -> (23.5, 21)
  line L1 (23.5, 21) -> (12.9938, 21)
  line L2 (12.9938, 21) -> (12.9938, 3)
  line L3 (12.9938, 3) -> (18.2469, 8.2531)
  line L4 (23.5, 3) -> (18.2469, 8.2531)
  line L5 (12.9938, 3) -> (23.5, 3)
  constraint coincident L2.end L3.start
  constraint coincident L0.start L4.start
  constraint perpendicular L3 L4
pattern_circular "C パターン1" [no effect]
sketch "スケッチ5" plane through (0, 0, 0) normal (1, 0, 0) x (0, 1, 0)
  line L0 (3, -16) -> (12, -16)
  line L1 (3, -16) -> (3, -10)
  line L2 (3, -10) -> (12, -10)
  line L3 (12, -10) -> (12, -16)
  constraint horizontal L0
  constraint perpendicular L0 L1
  constraint perpendicular L1 L2
  constraint perpendicular L0 L3
sketch "スケッチ8" plane through (0, 3, 0) normal (0, 1, 0) x (-1, 0, 0)
  line L0 (11.0273, 11.593) -> (15.4503, 16.016)
  line L1 (15.4503, 16.016) -> (16.016, 15.4503)
  line L2 (16.016, 15.4503) -> (11.593, 11.0273)
  arc A0 (11.593, 11.0273) -> (11.0273, 11.593) centre (0, 0) ccw
  arc A1 (4.5262, 15.3465) -> (3.7534, 15.5535) centre (0, 0) ccw
  line L3 (3.7534, 15.5535) -> (5.3724, 21.5954)
  line L4 (5.3724, 21.5954) -> (6.1451, 21.3883)
  line L5 (6.1451, 21.3883) -> (4.5262, 15.3465)
  arc A2 (-3.7534, 15.5535) -> (-4.5262, 15.3465) centre (0, 0) ccw
  line L6 (-4.5262, 15.3465) -> (-6.1451, 21.3883)
  line L7 (-6.1451, 21.3883) -> (-5.3724, 21.5954)
  line L8 (-5.3724, 21.5954) -> (-3.7534, 15.5535)
  arc A3 (-11.0273, 11.593) -> (-11.593, 11.0273) centre (0, 0) ccw
  line L9 (-11.593, 11.0273) -> (-16.016, 15.4503)
  line L10 (-16.016, 15.4503) -> (-15.4503, 16.016)
  line L11 (-15.4503, 16.016) -> (-11.0273, 11.593)
  arc A4 (-15.3465, 4.5262) -> (-15.5535, 3.7534) centre (0, 0) ccw
  line L12 (-15.5535, 3.7534) -> (-21.5954, 5.3724)
  line L13 (-21.5954, 5.3724) -> (-21.3883, 6.1451)
  line L14 (-21.3883, 6.1451) -> (-15.3465, 4.5262)
  arc A5 (-15.5535, -3.7534) -> (-15.3465, -4.5262) centre (0, 0) ccw
  line L15 (-15.3465, -4.5262) -> (-21.3883, -6.1451)
  line L16 (-21.3883, -6.1451) -> (-21.5954, -5.3724)
  line L17 (-21.5954, -5.3724) -> (-15.5535, -3.7534)
  arc A6 (-11.593, -11.0273) -> (-11.0273, -11.593) centre (0, 0) ccw
  line L18 (-11.0273, -11.593) -> (-15.4503, -16.016)
  line L19 (-15.4503, -16.016) -> (-16.016, -15.4503)
  line L20 (-16.016, -15.4503) -> (-11.593, -11.0273)
  circle A7 centre (-11.4718, 6.6232) radius 1.5
  circle A8 centre (0, 0) radius 10.7464
  circle A9 centre (-11.4718, -6.6232) radius 1.5
  circle A10 centre (11.4718, -6.6232) radius 1.5
  circle A11 centre (0, 13.2464) radius 1.5
  circle A12 centre (11.4718, 6.6232) radius 1.5
  circle A13 centre (0, -13.2464) radius 1.5
  line L21 (-3.7534, -15.5535) -> (-5.3724, -21.5954)
  line L22 (-5.3724, -21.5954) -> (-6.1451, -21.3883)
  line L23 (-6.1451, -21.3883) -> (-4.5262, -15.3465)
  arc A14 (-4.5262, -15.3465) -> (-3.7534, -15.5535) centre (0, 0) ccw
  line L24 (4.5262, -15.3465) -> (6.1451, -21.3883)
  line L25 (6.1451, -21.3883) -> (5.3724, -21.5954)
  line L26 (5.3724, -21.5954) -> (3.7534, -15.5535)
  arc A15 (3.7534, -15.5535) -> (4.5262, -15.3465) centre (0, 0) ccw
  line L27 (11.593, -11.0273) -> (16.016, -15.4503)
  line L28 (16.016, -15.4503) -> (15.4503, -16.016)
  line L29 (15.4503, -16.016) -> (11.0273, -11.593)
  arc A16 (11.0273, -11.593) -> (11.593, -11.0273) centre (0, 0) ccw
  line L30 (15.5535, -3.7534) -> (21.5954, -5.3724)
  line L31 (21.5954, -5.3724) -> (21.3883, -6.1451)
  line L32 (21.3883, -6.1451) -> (15.3465, -4.5262)
  arc A17 (15.3465, -4.5262) -> (15.5535, -3.7534) centre (0, 0) ccw
  line L33 (15.3465, 4.5262) -> (21.3883, 6.1451)
  line L34 (21.3883, 6.1451) -> (21.5954, 5.3724)
  line L35 (21.5954, 5.3724) -> (15.5535, 3.7534)
  arc A18 (15.5535, 3.7534) -> (15.3465, 4.5262) centre (0, 0) ccw
  arc A19 (9.8651, 12.4868) -> (11.2311, 12.8528) centre (10.3651, 13.3528) ccw
  line L36 (9.8651, 12.4868) -> (5.8814, 14.7868)
  arc A20 (5.5153, 16.1528) -> (5.8814, 14.7868) centre (6.3814, 15.6528) ccw
  line L37 (5.5153, 16.1528) -> (9.4969, 23.0491)
  arc A21 (9.4969, 23.0491) -> (9.2451, 23.765) centre (9.0639, 23.2991) ccw
  arc A22 (9.2451, 23.765) -> (3.876, 25.2037) centre (0, 0) ccw
  arc A23 (3.876, 25.2037) -> (3.3, 24.7095) centre (3.8, 24.7095) ccw
  line L38 (3.3, 24.7095) -> (3.3, 16.7464)
  arc A24 (2.3, 15.7464) -> (3.3, 16.7464) centre (2.3, 16.7464) ccw
  line L39 (2.3, 15.7464) -> (-2.3, 15.7464)
  arc A25 (-3.3, 16.7464) -> (-2.3, 15.7464) centre (-2.3, 16.7464) ccw
  line L40 (-3.3, 16.7464) -> (-3.3, 24.7095)
  arc A26 (-3.3, 24.7095) -> (-3.876, 25.2037) centre (-3.8, 24.7095) ccw
  arc A27 (-3.876, 25.2037) -> (-9.2451, 23.765) centre (0, 0) ccw
  arc A28 (-9.2451, 23.765) -> (-9.4969, 23.0491) centre (-9.0639, 23.2991) ccw
  line L41 (-9.4969, 23.0491) -> (-5.5153, 16.1528)
  arc A29 (-5.8814, 14.7868) -> (-5.5153, 16.1528) centre (-6.3814, 15.6528) ccw
  line L42 (-5.8814, 14.7868) -> (-9.8651, 12.4868)
  arc A30 (-11.2311, 12.8528) -> (-9.8651, 12.4868) centre (-10.3651, 13.3528) ccw
  line L43 (-11.2311, 12.8528) -> (-15.2126, 19.7491)
  arc A31 (-15.2126, 19.7491) -> (-15.9586, 19.889) centre (-15.6457, 19.4991) ccw
  arc A32 (-15.9586, 19.889) -> (-19.889, 15.9586) centre (0, 0) ccw
  arc A33 (-19.889, 15.9586) -> (-19.7491, 15.2126) centre (-19.4991, 15.6457) ccw
  line L44 (-19.7491, 15.2126) -> (-12.8528, 11.2311)
  arc A34 (-12.4868, 9.8651) -> (-12.8528, 11.2311) centre (-13.3528, 10.3651) ccw
  line L45 (-12.4868, 9.8651) -> (-14.7868, 5.8814)
  arc A35 (-16.1528, 5.5153) -> (-14.7868, 5.8814) centre (-15.6528, 6.3814) ccw
  line L46 (-16.1528, 5.5153) -> (-23.0491, 9.4969)
  arc A36 (-23.0491, 9.4969) -> (-23.765, 9.2451) centre (-23.2991, 9.0639) ccw
  arc A37 (-23.765, 9.2451) -> (-25.2037, 3.876) centre (0, 0) ccw
  arc A38 (-25.2037, 3.876) -> (-24.7095, 3.3) centre (-24.7095, 3.8) ccw
  line L47 (-24.7095, 3.3) -> (-16.7464, 3.3)
  arc A39 (-15.7464, 2.3) -> (-16.7464, 3.3) centre (-16.7464, 2.3) ccw
  line L48 (-15.7464, 2.3) -> (-15.7464, -2.3)
  arc A40 (-16.7464, -3.3) -> (-15.7464, -2.3) centre (-16.7464, -2.3) ccw
  line L49 (-16.7464, -3.3) -> (-24.7095, -3.3)
  arc A41 (-24.7095, -3.3) -> (-25.2037, -3.876) centre (-24.7095, -3.8) ccw
  arc A42 (-25.2037, -3.876) -> (-23.765, -9.2451) centre (0, 0) ccw
  arc A43 (-23.765, -9.2451) -> (-23.0491, -9.4969) centre (-23.2991, -9.0639) ccw
  line L50 (-23.0491, -9.4969) -> (-16.1528, -5.5153)
  arc A44 (-14.7868, -5.8814) -> (-16.1528, -5.5153) centre (-15.6528, -6.3814) ccw
  line L51 (-14.7868, -5.8814) -> (-12.4868, -9.8651)
  arc A45 (-12.8528, -11.2311) -> (-12.4868, -9.8651) centre (-13.3528, -10.3651) ccw
  line L52 (-12.8528, -11.2311) -> (-19.7491, -15.2126)
  arc A46 (-19.7491, -15.2126) -> (-19.889, -15.9586) centre (-19.4991, -15.6457) ccw
  arc A47 (-19.889, -15.9586) -> (-15.9586, -19.889) centre (0, 0) ccw
  arc A48 (-15.9586, -19.889) -> (-15.2126, -19.7491) centre (-15.6457, -19.4991) ccw
  line L53 (-15.2126, -19.7491) -> (-11.2311, -12.8528)
  arc A49 (-9.8651, -12.4868) -> (-11.2311, -12.8528) centre (-10.3651, -13.3528) ccw
  line L54 (-9.8651, -12.4868) -> (-5.8814, -14.7868)
  arc A50 (-5.5153, -16.1528) -> (-5.8814, -14.7868) centre (-6.3814, -15.6528) ccw
  line L55 (-5.5153, -16.1528) -> (-9.4969, -23.0491)
  arc A51 (-9.4969, -23.0491) -> (-9.2451, -23.765) centre (-9.0639, -23.2991) ccw
  arc A52 (-9.2451, -23.765) -> (-3.876, -25.2037) centre (0, 0) ccw
  arc A53 (-3.876, -25.2037) -> (-3.3, -24.7095) centre (-3.8, -24.7095) ccw
  line L56 (-3.3, -24.7095) -> (-3.3, -16.7464)
  arc A54 (-2.3, -15.7464) -> (-3.3, -16.7464) centre (-2.3, -16.7464) ccw
  line L57 (-2.3, -15.7464) -> (2.3, -15.7464)
  arc A55 (3.3, -16.7464) -> (2.3, -15.7464) centre (2.3, -16.7464) ccw
  line L58 (3.3, -16.7464) -> (3.3, -24.7095)
  arc A56 (3.3, -24.7095) -> (3.876, -25.2037) centre (3.8, -24.7095) ccw
  arc A57 (3.876, -25.2037) -> (9.2451, -23.765) centre (0, 0) ccw
  arc A58 (9.2451, -23.765) -> (9.4969, -23.0491) centre (9.0639, -23.2991) ccw
  line L59 (9.4969, -23.0491) -> (5.5153, -16.1528)
  arc A59 (5.8814, -14.7868) -> (5.5153, -16.1528) centre (6.3814, -15.6528) ccw
  line L60 (5.8814, -14.7868) -> (9.8651, -12.4868)
  arc A60 (11.2311, -12.8528) -> (9.8651, -12.4868) centre (10.3651, -13.3528) ccw
  line L61 (11.2311, -12.8528) -> (15.2126, -19.7491)
  arc A61 (15.2126, -19.7491) -> (15.9586, -19.889) centre (15.6457, -19.4991) ccw
  arc A62 (15.9586, -19.889) -> (19.889, -15.9586) centre (0, 0) ccw
  arc A63 (19.889, -15.9586) -> (19.7491, -15.2126) centre (19.4991, -15.6457) ccw
  line L62 (19.7491, -15.2126) -> (12.8528, -11.2311)
  arc A64 (12.4868, -9.8651) -> (12.8528, -11.2311) centre (13.3528, -10.3651) ccw
  line L63 (12.4868, -9.8651) -> (14.7868, -5.8814)
  arc A65 (16.1528, -5.5153) -> (14.7868, -5.8814) centre (15.6528, -6.3814) ccw
  line L64 (16.1528, -5.5153) -> (23.0491, -9.4969)
  arc A66 (23.0491, -9.4969) -> (23.765, -9.2451) centre (23.2991, -9.0639) ccw
  arc A67 (23.765, -9.2451) -> (25.2037, -3.876) centre (0, 0) ccw
  arc A68 (25.2037, -3.876) -> (24.7095, -3.3) centre (24.7095, -3.8) ccw
  line L65 (24.7095, -3.3) -> (16.7464, -3.3)
  arc A69 (15.7464, -2.3) -> (16.7464, -3.3) centre (16.7464, -2.3) ccw
  line L66 (15.7464, -2.3) -> (15.7464, 2.3)
  arc A70 (16.7464, 3.3) -> (15.7464, 2.3) centre (16.7464, 2.3) ccw
  line L67 (16.7464, 3.3) -> (24.7095, 3.3)
  arc A71 (24.7095, 3.3) -> (25.2037, 3.876) centre (24.7095, 3.8) ccw
  arc A72 (25.2037, 3.876) -> (23.765, 9.2451) centre (0, 0) ccw
  arc A73 (23.765, 9.2451) -> (23.0491, 9.4969) centre (23.2991, 9.0639) ccw
  line L68 (23.0491, 9.4969) -> (16.1528, 5.5153)
  arc A74 (14.7868, 5.8814) -> (16.1528, 5.5153) centre (15.6528, 6.3814) ccw
  line L69 (14.7868, 5.8814) -> (12.4868, 9.8651)
  arc A75 (12.8528, 11.2311) -> (12.4868, 9.8651) centre (13.3528, 10.3651) ccw
  line L70 (12.8528, 11.2311) -> (19.7491, 15.2126)
  arc A76 (19.7491, 15.2126) -> (19.889, 15.9586) centre (19.4991, 15.6457) ccw
  arc A77 (19.889, 15.9586) -> (15.9586, 19.889) centre (0, 0) ccw
  arc A78 (15.9586, 19.889) -> (15.2126, 19.7491) centre (15.6457, 19.4991) ccw
  line L71 (15.2126, 19.7491) -> (11.2311, 12.8528)
  circle A79 centre (0, 0) radius 15.7464
  circle A80 centre (0, -13.2464) radius 1.5
  circle A81 centre (11.4718, -6.6232) radius 1.5
  circle A82 centre (11.4718, 6.6232) radius 1.5
  circle A83 centre (0, 13.2464) radius 1.5
  circle A84 centre (-11.4718, 6.6232) radius 1.5
  circle A85 centre (-11.4718, -6.6232) radius 1.5
  line L72 (0, -4) -> (3.4641, -2)
  line L73 (3.4641, -2) -> (3.4641, 2)
  line L74 (3.4641, 2) -> (0, 4)
  line L75 (0, 4) -> (-3.4641, 2)
  line L76 (-3.4641, 2) -> (-3.4641, -2)
  line L77 (-3.4641, -2) -> (0, -4)
  dimension "d76" = 360
  constraint coincident A0.centre A1.centre
  constraint tangent L57 A79
  constraint concentric A13 A80
extrude "押し出し9" add sketch "スケッチ8" along normal blind 3 contours A8 | A79
move_body "移動11" bodies 1 to x (1, 0, 0) y (0, 1, 0) z (0, 0, 1) at (0, 0, -50)
sketch "スケッチ9" plane through (0, 6, 0) normal (0, 1, 0) x (-1, 0, 0)
  line L0 (0, -54) -> (-3.4641, -52)
  line L1 (-3.4641, -52) -> (-3.4641, -48)
  line L2 (-3.4641, -48) -> (0, -46)
  line L3 (0, -46) -> (3.4641, -48)
  line L4 (3.4641, -48) -> (3.4641, -52)
  line L5 (3.4641, -52) -> (0, -54)
  circle A0 centre (0, -36.7536) radius 1.5
  circle A1 centre (-11.4718, -43.3768) radius 1.5
  circle A2 centre (-11.4718, -56.6232) radius 1.5
  circle A3 centre (11.4718, -56.6232) radius 1.5
  circle A4 centre (11.4718, -43.3768) radius 1.5
  circle A5 centre (0, -63.2464) radius 1.5
  circle A6 centre (0, -50) radius 15.7464
  circle A7 centre (0, -50) radius 5.5
extrude "押し出し10" add sketch "スケッチ9" along normal blind 1.5 contours A7
sketch "スケッチ10" plane through (0, 7.5, 0) normal (0, 1, 0) x (-1, 0, 0)
  line L0 (3.4641, -48) -> (3.4641, -52)
  line L1 (3.4641, -52) -> (0, -54)
  line L2 (0, -54) -> (-3.4641, -52)
  line L3 (-3.4641, -52) -> (-3.4641, -48)
  line L4 (-3.4641, -48) -> (0, -46)
  line L5 (0, -46) -> (3.4641, -48)
  circle A0 centre (0, -50) radius 5.5
  circle A1 centre (0, -50) radius 5.5
  constraint concentric A0 A1
extrude "押し出し11" add sketch "スケッチ10" along normal blind 3 contours L0 L1 L2 L3 L4 L5 | A0 A1
sketch "スケッチ11" plane through (0, 10.5, 0) normal (0, 1, 0) x (-1, 0, 0)
  circle A0 centre (0, -50) radius 5.5
  circle A1 centre (0, -50) radius 1.5
  dimension "d88" = 3
  constraint concentric A0 A1
  measures "d88" diameter of A1
extrude "押し出し12" cut sketch "スケッチ11" against normal blind 45 contours A1
sketch "スケッチ12" plane through (0, 0, 0) normal (1, 0, 0) x (0, 1, 0)
  line L0 (6, -61) -> (10.5, -55.5)
  line L1 (10.5, -55.5) -> (6, -55.5)
  line L2 (6, -55.5) -> (6, -61)
  line L3 (11, -50) -> (13, -50)
  constraint horizontal L1
  constraint perpendicular L1 L2
  constraint horizontal L3
revolve "回転2" add sketch "スケッチ12" angle 360 about axis through (0, 11, -50) along (0, 1, 0)
sketch "スケッチ13" plane through (0, 3, 0) normal (0, -1, 0) x (1, 0, 0)
  line L0 (3.4641, -52) -> (0, -54)
  line L1 (0, -54) -> (-3.4641, -52)
  line L2 (-3.4641, -52) -> (-3.4641, -48)
  line L3 (-3.4641, -48) -> (0, -46)
  line L4 (0, -46) -> (3.4641, -48)
  line L5 (3.4641, -48) -> (3.4641, -52)
  circle A0 centre (0, -36.7536) radius 1.5
  circle A1 centre (11.4718, -43.3768) radius 1.5
  circle A2 centre (11.4718, -56.6232) radius 1.5
  circle A3 centre (-11.4718, -56.6232) radius 1.5
  circle A4 centre (-11.4718, -43.3768) radius 1.5
  circle A5 centre (0, -63.2464) radius 1.5
  circle A6 centre (0, -50) radius 15.7464
  line L6 (0, -45.9) -> (-3.5507, -47.95)
  line L7 (-3.5507, -47.95) -> (-3.5507, -52.05)
  line L8 (-3.5507, -52.05) -> (0, -54.1)
  line L9 (0, -54.1) -> (3.5507, -52.05)
  line L10 (3.5507, -52.05) -> (3.5507, -47.95)
  line L11 (3.5507, -47.95) -> (0, -45.9)
  point P0 (0, -50)
  dimension "d92" = 4.1
  constraint coincident P0 A6.centre
  measures "d92" distance of L6.start P0
extrude "押し出し13" cut sketch "スケッチ13" against normal blind 4.5 contours L6 L7 L8 L9 L10 L11
move_body "移動14" bodies 1 to x (1, 0, 0) y (0, 1, 0) z (0, 0, 1) at (0, 0, 50)
move_body "移動15" bodies 1 to x (1, 0, 0) y (0, 1, 0) z (0, 0, 1) at (62, 4, 0)
move_body "移動16" bodies 1 to x (1, 0, 0) y (0, 1, 0) z (0, 0, 1) at (-62, -7, 0)
